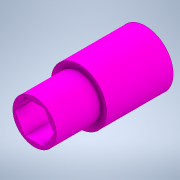
# Autodesk Inventor part: 3_8x5_8x3_4-hexBearingEndCap
Saved by Autodesk Inventor 2021.2 (Build 252289000, 289)
## iProperties
Created: 2020-11-08
Part Number: 3_8x5_8x3_4-hexBearingEndCap
Material: PC/ABS Plastic
Document SubType Name: Modeling
Designer: robst
Density: 0.357273 g/cm^3
Appearance: Magenta
Author: robst
Autodesk Inventor part; units mm, degrees
ref_plane "YZ Plane" through (0, 0, 0) normal (1, 0, 0) x (0, 1, 0)
ref_plane "XZ Plane" through (0, 0, 0) normal (0, 1, 0) x (-1, 0, 0)
ref_plane "XY Plane" through (0, 0, 0) normal (0, 0, 1) x (1, 0, 0)
sketch "Sketch1" plane through (0, 0, 0) normal (0, 0, 1) x (1, 0, 0)
  line L0 (2.7496, 4.7625) -> (5.4993, 0)
  line L1 (5.4993, 0) -> (2.7496, -4.7625)
  line L2 (2.7496, -4.7625) -> (-2.7496, -4.7625)
  line L3 (-2.7496, -4.7625) -> (-5.4993, 0)
  line L4 (-5.4993, 0) -> (-2.7496, 4.7625)
  line L5 (-2.7496, 4.7625) -> (2.7496, 4.7625)
  circle A0 centre (0, 0) radius 7.9375
  circle A1 centre (0, 0) radius 5.4993 construction
  dimension "d0" = 9.525
  dimension "d2" = 15.875
  dimension "d3" = 2.4382
  constraints: 12 end point, 3 coincident, 1 centre point, 1 horizontal, 1 horizontal alignment, 15 other
  measures "d0" distance between parallel lines of L2 L5
  measures "d2" diameter of A0
extrude "Extrusion1" add sketch "Sketch1" against normal blind 19.05
thicken "Thicken Hex" operation add thickness 0.127 both sides no extend neighbours yes toward (-0.8660254, 0.5, 0) faces at (-4.5827, 1.5875, -6.35) (-3.6662, -3.175, -6.35) (0.9165, -4.7625, -6.35) (-0.9165, 4.7625, -6.35) (3.6662, 3.175, -6.35) (4.5827, -1.5875, -6.35)
sketch "Sketch3" plane through (0, 0, 0) normal (0, 0, 1) x (1, 0, 0)
  line L0 (5.6459, 0) -> (2.823, -4.8895)
  line L1 (2.823, -4.8895) -> (-2.823, -4.8895)
  line L2 (-2.823, -4.8895) -> (-5.6459, 0)
  line L3 (-5.6459, 0) -> (-2.823, 4.8895)
  line L4 (-2.823, 4.8895) -> (2.823, 4.8895)
  line L5 (2.823, 4.8895) -> (5.6459, 0)
  line L6 (2.823, 4.8895) -> (5.6459, 0) projected
  circle A0 centre (0, 0) radius 6.35
  dimension "d10" = 12.7
  constraints: 12 end point, 2 coincident, 1 centre point, 1 collinear, 1 horizontal, 13 other
  measures "d10" diameter of A0
extrude "Extrusion2" add sketch "Sketch3" along normal blind 12.7
thicken "Thicken2" operation add thickness 0.127 both sides no extend neighbours yes toward (-0.9967573, 0.0804666, 0) faces at (6.3294, -0.511, 8.4667)
equation "\"d0\" = hexSize"
equation "\"d2\" = exteriorDiameter"
equation "\"d4\" = length"
equation "\"d6\" = printSpacing"
equation "\"d7\" = printSpacing"
equation "\"d10\" = baseBushingDiameter"
equation "\"d8\" = baseBushingLength"
equation "\"d11\" = printSpacing"
equation "\"d12\" = printSpacing"
equation "\"hexSize\" = 9.525"
equation "\"exteriorDiameter\" = 15.875"
equation "\"length\" = 19.05"
equation "\"printSpacing\" = 0.127"
equation "\"baseBushingDiameter\" = 12.7"
equation "\"baseBushingLength\" = 12.7"
body "Solid1"
